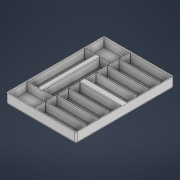
# Autodesk Inventor part: Pocker lower half
Saved by Autodesk Inventor 2022 (Build 260153000, 153)
## iProperties
Created: 2021-05-24
Part Number: Pocker lower half
Material: Aluminum 6061-AHC
Document SubType Name: Modeling
Designer: Albert L Tomberg
Density: 2.7 g/cm^3
Appearance: Aluminum - Polished
Author: Albert L Tomberg
Autodesk Inventor part; units mm, degrees
ref_plane "YZ Plane" through (0, 0, 0) normal (1, 0, 0) x (0, 1, 0)
ref_plane "XZ Plane" through (0, 0, 0) normal (0, 1, 0) x (-1, 0, 0)
ref_plane "XY Plane" through (0, 0, 0) normal (0, 0, 1) x (1, 0, 0)
sketch "Sketch1" plane through (0, 0, 0) normal (0, 1, 0) x (-1, 0, 0)
  line L0 (0, 0) -> (250, 0)
  line L1 (250, 0) -> (250, -350)
  line L2 (250, -350) -> (0, -350)
  line L3 (0, -350) -> (0, 0)
  dimension "d0" = 250
  dimension "d1" = 350
  constraints: 8 end point, 2 parallel, 1 horizontal, 1 perpendicular
  measures "d0" distance of L1.end L2.end
  measures "d1" distance of L0.end L1.end
extrude "Extrusion1" add sketch "Sketch1" along normal blind 35
sketch "Sketch2" plane through (0, 35, 0) normal (0, 1, 0) x (1, 0, 0)
  line L0 (-5, 5) -> (-245, 5)
  line L1 (-245, 5) -> (-245, 345)
  line L2 (-245, 345) -> (-5, 345)
  line L3 (-5, 345) -> (-5, 5)
  line L4 (-245, 70) -> (-155, 70)
  line L5 (-155, 70) -> (-155, 5)
  line L6 (-245, 280) -> (-155, 280)
  line L7 (-155, 280) -> (-155, 345)
  line L8 (-250, 350) -> (-250, 0) projected
  line L9 (-250, 0) -> (0, 0) projected
  line L10 (-245, 75) -> (-155, 75)
  line L11 (-150, 5) -> (-150, 41)
  line L12 (-150, 41) -> (-5, 41)
  line L13 (-150, 41) -> (-150, 46)
  line L14 (-150, 46) -> (-5, 46)
  line L15 (-150, 46) -> (-150, 82)
  line L16 (-150, 46) -> (-114, 46) construction
  line L17 (-150, 82) -> (-5, 82)
  line L18 (-150, 345) -> (-150, 309)
  line L19 (-150, 309) -> (-5, 309)
  line L20 (-150, 309) -> (-150, 304)
  line L21 (-150, 304) -> (-5, 304)
  line L22 (-150, 304) -> (-150, 268)
  line L23 (-150, 268) -> (-5, 268)
  line L24 (-245, 275) -> (-155, 275)
  line L25 (-155, 275) -> (-155, 75)
  line L26 (-150, 82) -> (-150, 87)
  line L27 (-150, 87) -> (-5, 87)
  line L28 (-150, 87) -> (-150, 123)
  line L29 (-150, 123) -> (-5, 123)
  line L30 (-150, 268) -> (-150, 263)
  line L31 (-150, 263) -> (-5, 263)
  line L32 (-150, 263) -> (-150, 227)
  line L33 (-150, 227) -> (-5, 227)
  line L34 (-150, 227) -> (-150, 222)
  line L35 (-150, 222) -> (-5, 222)
  line L36 (-150, 123) -> (-150, 128)
  line L37 (-150, 128) -> (-5, 128)
  line L38 (-150, 128) -> (-150, 164)
  line L39 (-150, 164) -> (-5, 164)
  line L40 (-150, 222) -> (-150, 186)
  line L41 (-150, 186) -> (-5, 186)
  line L42 (-245, 75) -> (-209, 75)
  line L43 (-209, 75) -> (-209, 275)
  line L44 (-155, 75) -> (-191, 75)
  line L45 (-191, 75) -> (-191, 275)
  dimension "d4" = 240
  dimension "d5" = 340
  dimension "d6" = 90
  dimension "d7" = 90
  dimension "d10" = 65
  dimension "d11" = 5
  dimension "d12" = 5
  dimension "d20" = 90
  dimension "d21" = 36
  dimension "d22" = 5
  dimension "d23" = 36
  dimension "d24" = 90
  dimension "d25" = 36
  dimension "d26" = 5
  dimension "d27" = 36
  dimension "d28" = 5
  dimension "d29" = 36
  dimension "d30" = 5
  dimension "d31" = 36
  dimension "d32" = 5
  dimension "d33" = 5
  dimension "d34" = 36
  dimension "d35" = 36
  dimension "d36" = 36
  dimension "d37" = 36
  dimension "d38" = 200
  dimension "d39" = 5
  dimension "d40" = 18
  dimension "d41" = 36
  dimension "d42" = 145
  dimension "d43" = 145
  constraints: 86 end point, 25 point on line, 15 horizontal, 12 perpendicular, 1 parallel, 1 vertical, 17 other
  measures "d4" distance of L1.end L2.end
  measures "d5" distance of L0.end L1.end
  measures "d6" distance of L4.start L4.end
  measures "d7" distance of L6.start L6.end
  measures "d10" distance between parallel lines of L0 L4
  measures "d11" distance between parallel lines of L8 L1
  measures "d12" distance between parallel lines of L9 L0
  measures "d20" angle of L7 L6
  measures "d21" distance of L11.start L11.end
  measures "d22" distance of L11.end L13.end
  measures "d23" distance of L13.end L15.end
  measures "d24" angle of L16 L15
  measures "d25" distance of L18.start L18.end
  measures "d26" distance of L18.end L20.end
  measures "d27" distance of L20.end L22.end
  measures "d28" distance of L15.end L26.end
  measures "d29" distance of L26.end L28.end
  measures "d30" distance of L22.end L30.end
  measures "d31" distance of L30.end L32.end
  measures "d32" distance of L32.end L34.end
  measures "d33" distance of L28.end L36.end
  measures "d34" distance of L36.end L38.end
  measures "d35" distance of L34.end L40.end
  measures "d36" distance of L10.start L42.end
  measures "d37" distance of L10.end L44.end
  measures "d38" distance between parallel lines of L24 L10
  measures "d39" distance between parallel lines of L4 L10
  measures "d40" distance between parallel lines of L43 L45
  measures "d41" distance between parallel lines of L39 L37
  measures "d42" distance of L28.end L29.end
  measures "d43" distance of L40.end L41.end
extrude "Extrusion2" cut sketch "Sketch2" against normal blind 30 contours L0 L11 L12 L3 | L0 L1 L4 L5 | L14 L15 L17 L3 | L27 L28 L29 L3 | L1 L24 L43 L10 | L37 L38 L39 L3 | L1 L2 L7 L6 | L45 L24 L25 L10 | L41 L40 L35 L3 | L2 L3 L19 L18 | L33 L32 L31 L3 | L21 L3 L23 L22
fillet "Fillet1" radius 5 8 edges at (-125, 0, 0) (0, 17.5, 0) (0, 0, -175) (0, 17.5, -350) (-125, 0, -350) (-250, 17.5, -350) (-250, 0, -175) (-250, 17.5, 0)
fillet "Fillet2" radius 2 7 edges at (-155, 20, -345) (-155, 20, -70) (-245, 20, -345) (-245, 20, -280) (-245, 20, -5) (-245, 20, -70) (-155, 20, -5)
fillet "Fillet3" radius 2 1 edges at (-155, 20, -280)
fillet "Fillet5" radius 2 56 edges at (-150, 35, -23) (-77.5, 35, -5) (-5, 35, -23) (-77.5, 35, -41) (-77.5, 35, -46) (-5, 35, -64) (-77.5, 35, -82) (-150, 35, -64) (-77.5, 35, -87) (-150, 35, -105) (-77.5, 35, -123) (-5, 35, -105) (-5, 35, -146) (-77.5, 35, -164) (-77.5, 35, -128) (-150, 35, -146) (-77.5, 35, -186) (-150, 35, -204) (-77.5, 35, -222) (-5, 35, -204) (-77.5, 35, -263) (-150, 35, -245) (-77.5, 35, -227) (-5, 35, -245) (-5, 35, -286) (-77.5, 35, -304) (-150, 35, -286) (-77.5, 35, -268) (-77.5, 35, -345) (-150, 35, -327) (-77.5, 35, -309) (-5, 35, -327) (-155, 35, -175) (-173, 35, -75) (-191, 35, -175) (-173, 35, -275) (-209, 35, -175) (-245, 35, -175) (-227, 35, -275) (-227, 35, -75) (-155.5858, 35, -69.4142) (-155, 35, -37.5) (-155.5858, 35, -5.5858) (-200, 35, -5) (-244.4142, 35, -5.5858) (-245, 35, -37.5) (-244.4142, 35, -69.4142) (-200, 35, -70) (-244.4142, 35, -280.5858) (-245, 35, -312.5) (-244.4142, 35, -344.4142) (-200, 35, -345) (-155.5858, 35, -344.4142) (-155, 35, -312.5) (-155.5858, 35, -280.5858) (-200, 35, -280)
fillet "Fillet6" radius 1 120 edges at (-150, 5, -23) (-150, 5, -64) (-150, 5, -105) (-150, 5, -146) (-150, 5, -204) (-150, 5, -245) (-150, 5, -286) (-150, 5, -327) (-77.5, 5, -345) (-77.5, 5, -304) (-77.5, 5, -268) (-77.5, 5, -263) (-77.5, 5, -227) (-77.5, 5, -222) (-77.5, 5, -186) (-77.5, 5, -164) (-77.5, 5, -128) (-77.5, 5, -123) (-77.5, 5, -87) (-77.5, 5, -82) (-77.5, 5, -46) (-77.5, 5, -41) (-77.5, 5, -5) (-5, 5, -23) (-5, 5, -64) (-5, 5, -105) (-5, 5, -146) (-5, 5, -204) (-5, 5, -245) (-5, 5, -286) (-5, 5, -327) (-77.5, 5, -309) (-150.5858, 34.4142, -164.5858) (-150, 19, -164) (-150.5858, 34.4142, -127.4142) (-150, 19, -128) (-4.4142, 34.4142, -164.5858) (-5, 19, -164) (-4.4142, 34.4142, -127.4142) (-5, 19, -128) (-4.4142, 34.4142, -123.5858) (-5, 19, -123) (-4.4142, 34.4142, -86.4142) (-5, 19, -87) (-4.4142, 34.4142, -82.5858) (-5, 19, -82) (-150.5858, 34.4142, -123.5858) (-150, 19, -123) (-150.5858, 34.4142, -86.4142) (-150, 19, -87) (-150.5858, 34.4142, -82.5858) (-150, 19, -82) (-150.5858, 34.4142, -45.4142) (-150, 19, -46) (-150.5858, 34.4142, -41.5858) (-150, 19, -41) (-150.5858, 34.4142, -4.4142) (-150, 19, -5) (-4.4142, 34.4142, -4.4142) (-5, 19, -5) (-4.4142, 34.4142, -41.5858) (-5, 19, -41) (-4.4142, 34.4142, -45.4142) (-5, 19, -46) (-4.4142, 34.4142, -185.4142) (-5, 19, -186) (-4.4142, 34.4142, -222.5858) (-5, 19, -222) (-4.4142, 34.4142, -226.4142) (-5, 19, -227) (-4.4142, 34.4142, -263.5858) (-5, 19, -263) (-4.4142, 34.4142, -267.4142) (-5, 19, -268) (-4.4142, 34.4142, -304.5858) (-5, 19, -304) (-4.4142, 34.4142, -308.4142) (-5, 19, -309) (-4.4142, 34.4142, -345.5858) (-5, 19, -345) (-150.5858, 34.4142, -345.5858) (-150, 19, -345) (-150.5858, 34.4142, -308.4142) (-150, 19, -309) (-150.5858, 34.4142, -304.5858) (-150, 19, -304) (-150.5858, 34.4142, -267.4142) (-150, 19, -268) (-150.5858, 34.4142, -263.5858) (-150, 19, -263) (-150.5858, 34.4142, -226.4142) (-150, 19, -227) (-150.5858, 34.4142, -222.5858) (-150, 19, -222) (-150.5858, 34.4142, -185.4142) (-150, 19, -186) (-155, 5, -175) (-173, 5, -275) (-154.4142, 34.4142, -275.5858) (-155, 19, -275) (-191, 5, -175) (-191.5858, 34.4142, -275.5858) (-191, 19, -275) (-154.4142, 34.4142, -74.4142) (-155, 19, -75) (-173, 5, -75) (-191.5858, 34.4142, -74.4142) (-191, 19, -75) (-209, 5, -175) (-208.4142, 34.4142, -275.5858) (-209, 19, -275) (-245.5858, 34.4142, -275.5858) (-245, 19, -275) (-227, 5, -275) (-245, 5, -175) (-245.5858, 34.4142, -74.4142) (-245, 19, -75) (-227, 5, -75) (-208.4142, 34.4142, -74.4142) (-209, 19, -75)
body "Solid1"
